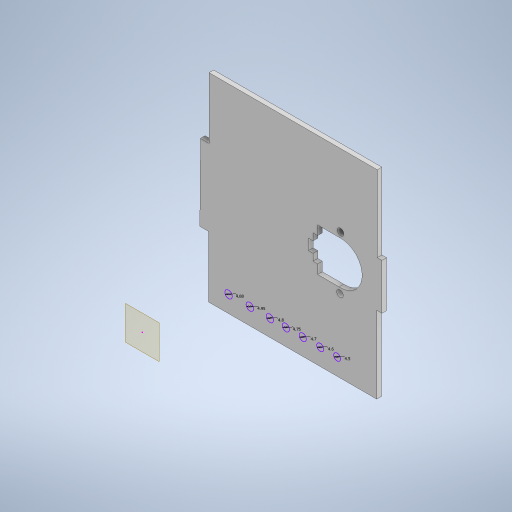
# Autodesk Inventor part: MotorMountPlate
Saved by Autodesk Inventor 2023 (Build 270158000, 158)
## iProperties
Created: 2022-10-06
Part Number: MotorMountPlate
Material: Generic
Document SubType Name: Modeling
Designer: digge
Density: 1 g/cm^3
Appearance: Default
Author: digge
Autodesk Inventor part; units mm, degrees
ref_plane "YZ Plane" through (0, 0, 0) normal (1, 0, 0) x (0, 1, 0)
ref_plane "XZ Plane" through (0, 0, 0) normal (0, 1, 0) x (-1, 0, 0)
ref_plane "XY Plane" through (0, 0, 0) normal (0, 0, 1) x (1, 0, 0)
sketch "Sketch2" plane through (0, 0, 0) normal (0, 0, 1) x (1, 0, 0)
  line L0 (130.6479, 118.1756) -> (130.6479, 90.1756)
  circle A0 centre (129.6479, 104.1756) radius 14.0357
  line L1 (39.8344, 104.1756) -> (88.8344, 104.1756)
  line L2 (130.6479, 90.1756) -> (114.6267, 90.1756)
  line L3 (114.6267, 118.1756) -> (130.6479, 118.1756)
  arc A1 (143.6267, 102.9137) -> (130.6479, 118.1756) centre (129.6479, 104.1756) ccw
  arc A2 (130.6479, 90.1756) -> (143.6267, 102.9137) centre (129.6479, 104.1756) ccw
  line L4 (130.6479, 90.1756) -> (114.6267, 90.1756)
  line L5 (114.6267, 118.1756) -> (130.6479, 118.1756)
  line L6 (153.6267, 168.8936) -> (43.6267, 168.8936)
  line L7 (43.6267, 168.8936) -> (43.6267, 128.8928)
  line L8 (43.6267, 128.8928) -> (38.0267, 128.8928)
  line L9 (38.0267, 128.8928) -> (37.642, 78.8943)
  line L10 (37.642, 78.8943) -> (43.2388, 78.8943)
  line L11 (43.2388, 78.8943) -> (43.2388, 38.8936)
  line L12 (43.2388, 38.8936) -> (153.2388, 38.8936)
  line L13 (153.2388, 38.8936) -> (153.2388, 89.1756)
  line L14 (153.6267, 119.1756) -> (153.6267, 168.8936)
  line L15 (114.6267, 118.1756) -> (114.6267, 112.1756)
  line L16 (114.6267, 112.1756) -> (111.6267, 112.1756)
  line L17 (111.6267, 112.1756) -> (111.6267, 107.6756)
  line L18 (111.6267, 107.6756) -> (108.6267, 107.6756)
  line L19 (108.6267, 107.6756) -> (108.6267, 100.6756)
  line L20 (108.6267, 100.6756) -> (111.6267, 100.6756)
  line L21 (111.6267, 100.6756) -> (111.6267, 96.1756)
  line L22 (111.6267, 96.1756) -> (114.6267, 96.1756)
  line L23 (114.6267, 96.1756) -> (114.6267, 90.1756)
  line L24 (153.6267, 119.1756) -> (156.6267, 119.1756)
  line L25 (156.6267, 119.1756) -> (156.6267, 89.1756)
  line L26 (156.6267, 89.1756) -> (153.2388, 89.1756)
  circle A3 centre (129.2388, 86.6756) radius 2.15
  circle A4 centre (129.6267, 121.6756) radius 2.15
  point P0 (0, 0)
  point P1 (128.6479, 118.1756)
  point P2 (128.6479, 90.1756)
  point P3 (122.6373, 90.1756)
  point P4 (122.6373, 118.1756)
  dimension "d0" = 50
  dimension "d1" = 130
  dimension "d2" = 28.0713
  dimension "d3" = 7
  dimension "d4" = 3
  dimension "d5" = 6
  dimension "d6" = 6
  dimension "d7" = 110
  dimension "d8" = 110
  dimension "d9" = 5.6
  dimension "d10" = 3
  dimension "d11" = 32
  dimension "d13" = 10
  dimension "d14" = 30
  dimension "d15" = 3
  dimension "d18" = 28
  dimension "d28" = 4.3
  dimension "d29" = 24
  dimension "d30" = 3.5
  dimension "d31" = 4.3
  dimension "d32" = 24
  dimension "d33" = 3.5
  constraints: 54 end point, 9 perpendicular, 7 point on circle, 5 centre point, 5 horizontal, 4 parallel, 4 vertical, 3 equal length, 2 midpoint, 1 point on line, 2 other
  measures "d0" distance of L8.end L9.end
  measures "d1" distance between parallel lines of L6 L12
  measures "d2" diameter of A0
  measures "d3" distance of L18.end L19.end
  measures "d4" distance of L17.end L18.end
  measures "d5" distance of L3.start L15.end
  measures "d6" distance of L22.end L2.end
  measures "d7" distance of L6.start L6.end
  measures "d8" distance of L11.end L12.end
  measures "d9" distance of L7.end L8.end
  measures "d10" distance of L15.end L16.end
  measures "d11" distance from line of A1.start L17
  measures "d13" distance from line of L14 A1.start
  measures "d14" distance of L24.end L25.end
  measures "d15" distance of L14.start L24.end
  measures "d18" distance between parallel lines of L2 L3
  measures "d28" diameter of A3
  measures "d29" distance from line of A3.centre L13
  measures "d30" vertical distance of point (122.637, 90.176) A3.centre
  measures "d31" diameter of A4
  measures "d32" distance from line of L14 A4.centre
  measures "d33" vertical distance of point (122.637, 118.176) A4.centre
ref_plane "Work Plane1" through (0, 0, 3) normal (0, 0, 1) x (1, 0, 0)
sketch "Sketch3" plane through (0, 0, 3) normal (0, 0, 1) x (1, 0, 0)
  circle A0 centre (56.2766, 49.819) radius 2.44
  circle A1 centre (70.2268, 49.819) radius 2.475
  circle A2 centre (83.2893, 49.819) radius 2.4
  circle A3 centre (93.7333, 49.819) radius 2.375
  circle A4 centre (104.7615, 49.819) radius 2.35
  circle A5 centre (116.1801, 49.819) radius 2.3
  circle A6 centre (127.2083, 49.819) radius 2.25
  point P0 (0, 0)
  dimension "d19" = 4.88
  dimension "d20" = 4.95
  dimension "d21" = 4.8
  dimension "d24" = 4.75
  dimension "d25" = 4.7
  dimension "d26" = 4.6
  dimension "d27" = 4.5
  constraints: 7 centre point
  measures "d19" diameter of A0
  measures "d20" diameter of A1
  measures "d21" diameter of A2
  measures "d24" diameter of A3
  measures "d25" diameter of A4
  measures "d26" diameter of A5
  measures "d27" diameter of A6
extrude "Extrusion3" add sketch "Sketch2" along normal blind 3
body "Solid2"
